Autodesk Fusion 360 part; units mm, degrees
(part 4 of 6)
sketch "USB clamp fixed housing post sketch" plane through (0, 0, 37.2) normal (0, 0, 1) x (1, 0, 0) in component "01 Tapered printed housing"
  circle A0 centre (70, 16) radius 4.3
  dimension "d1306" = 70
  dimension "d1307" = 16
  dimension "d1308" = 4.3
  measures "d1306" horizontal distance of origin A0.centre
  measures "d1307" vertical distance of origin A0.centre
  measures "d1308" radius of A0
extrude "USB clamp fixed housing post" add sketch "USB clamp fixed housing post sketch" along normal blind 6 bodies 1 in component "01 Tapered printed housing"
ref_plane "WorkPlane33" through (0, 0, 39.2) normal (0, 0, 1) x (1, 0, 0) in component "01 Tapered printed housing"
sketch "USB clamp insert pilot reference sketch" plane through (0, 0, 39.2) normal (0, 0, 1) x (1, 0, 0) in component "01 Tapered printed housing"
  circle A0 centre (69.3, 16) radius 1.6
  dimension "d1313" = 69.3
  dimension "d1314" = 16
  dimension "d1315" = 1.6
  measures "d1313" horizontal distance of origin A0.centre
  measures "d1314" vertical distance of origin A0.centre
  measures "d1315" radius of A0
extrude "USB clamp insert pilot reference" cut sketch "USB clamp insert pilot reference sketch" along normal blind 4.1 bodies 1 in component "01 Tapered printed housing"
ref_plane "WorkPlane1" through (0, 0, 43.2) normal (0, 0, 1) x (1, 0, 0) in component "USB — removable rear housing clamp"
sketch "USB rear clamp strap sketch" plane through (0, 0, 43.2) normal (0, 0, 1) x (1, 0, 0) in component "USB — removable rear housing clamp"
  line L0 (65.7, 8.5) -> (72.4, 8.5)
  line L1 (72.4, 8.5) -> (72.4, 20.3)
  line L2 (72.4, 20.3) -> (65.7, 20.3)
  line L3 (65.7, 20.3) -> (65.7, 8.5)
  dimension "d1320" = 65.7
  dimension "d1321" = 8.5
  dimension "d1322" = 6.7
  dimension "d1323" = 11.8
  constraint horizontal L0
  constraint vertical L1
  constraint horizontal L2
  constraint vertical L3
  measures "d1320" horizontal distance of origin L0.start
  measures "d1321" vertical distance of origin L0.start
  measures "d1322" horizontal distance of L0.start L0.end
  measures "d1323" vertical distance of L0.end L1.end
extrude "USB rear clamp strap" add sketch "USB rear clamp strap sketch" along normal blind 2 separate body makes body 61 in component "USB — removable rear housing clamp"
ref_plane "WorkPlane2" through (0, 0, 35) normal (0, 0, 1) x (1, 0, 0) in component "USB — removable rear housing clamp"
sketch "USB inward stop and offset stalk sketch" plane through (0, 0, 35) normal (0, 0, 1) x (1, 0, 0) in component "USB — removable rear housing clamp"
  line L0 (68.4, 8.5) -> (70.4, 8.5)
  line L1 (70.4, 8.5) -> (70.4, 10.5)
  line L2 (70.4, 10.5) -> (68.4, 10.5)
  line L3 (68.4, 10.5) -> (68.4, 8.5)
  dimension "d1328" = 68.4
  dimension "d1329" = 8.5
  dimension "d1330" = 2
  dimension "d1331" = 2
  constraint horizontal L0
  constraint vertical L1
  constraint horizontal L2
  constraint vertical L3
  measures "d1328" horizontal distance of origin L0.start
  measures "d1329" vertical distance of origin L0.start
  measures "d1330" horizontal distance of L0.start L0.end
  measures "d1331" vertical distance of L0.end L1.end
extrude "USB inward stop and offset stalk" add sketch "USB inward stop and offset stalk sketch" along normal blind 8.3 bodies 61 in component "USB — removable rear housing clamp"
ref_plane "WorkPlane3" through (0, 0, 43.1) normal (0, 0, 1) x (1, 0, 0) in component "USB — removable rear housing clamp"
sketch "USB clamp M2 clearance sketch" plane through (0, 0, 43.1) normal (0, 0, 1) x (1, 0, 0) in component "USB — removable rear housing clamp"
  circle A0 centre (69.3, 16) radius 1.1
  dimension "d1336" = 69.3
  dimension "d1337" = 16
  dimension "d1338" = 1.1
  measures "d1336" horizontal distance of origin A0.centre
  measures "d1337" vertical distance of origin A0.centre
  measures "d1338" radius of A0
extrude "USB clamp M2 clearance" cut sketch "USB clamp M2 clearance sketch" along normal blind 2.2 bodies 61 in component "USB — removable rear housing clamp"
ref_plane "WorkPlane1" through (0, 0, 48.8) normal (0, 0, 1) x (1, 0, 0) in component "Chamber / removable internal lid"
sketch "Internal L lid sketch" plane through (0, 0, 48.8) normal (0, 0, 1) x (1, 0, 0) in component "Chamber / removable internal lid"
  line L0 (2.9, 87) -> (72.1, 87)
  line L1 (72.1, 87) -> (72.1, 122.1)
  line L2 (72.1, 122.1) -> (2.9, 122.1)
  line L3 (2.9, 122.1) -> (2.9, 87)
  dimension "d1609" = 2.9
  dimension "d1610" = 87
  constraint horizontal L0
  constraint vertical L1
  constraint horizontal L2
  constraint vertical L3
  measures "d1609" horizontal distance of origin L0.start
  measures "d1610" vertical distance of origin L0.start
extrude "Internal L lid" add sketch "Internal L lid sketch" along normal blind 2 separate body makes body 62 in component "Chamber / removable internal lid"
ref_plane "WorkPlane2" through (0, 0, 48.8) normal (0, 0, 1) x (1, 0, 0) in component "Chamber / removable internal lid"
sketch "Internal L lid side column sketch" plane through (0, 0, 48.8) normal (0, 0, 1) x (1, 0, 0) in component "Chamber / removable internal lid"
  line L0 (45.6, 30) -> (72.1, 30)
  line L1 (72.1, 30) -> (72.1, 122.1)
  line L2 (72.1, 122.1) -> (45.6, 122.1)
  line L3 (45.6, 122.1) -> (45.6, 30)
  dimension "d1617" = 45.6
  dimension "d1618" = 30
  constraint horizontal L0
  constraint vertical L1
  constraint horizontal L2
  constraint vertical L3
  measures "d1617" horizontal distance of origin L0.start
  measures "d1618" vertical distance of origin L0.start
extrude "Internal L lid side column" add sketch "Internal L lid side column sketch" along normal blind 2 bodies 62 in component "Chamber / removable internal lid"
fillet "Lid housing-clearance top rounds" radius 3.1 2 edges at (2.9, 122.1, 49.8) (72.1, 122.1, 49.8) on bodies 62 in component "Chamber / removable internal lid"
ref_plane "WorkPlane3" through (0, 0, 15.5) normal (0, 0, 1) x (1, 0, 0) in component "Chamber / removable internal lid"
sketch "Lid upper M3 post clearance sketch" plane through (0, 0, 15.5) normal (0, 0, 1) x (1, 0, 0) in component "Chamber / removable internal lid"
  circle A0 centre (6, 119) radius 4.5
  dimension "d1627" = 6
  dimension "d1628" = 119
  dimension "d1629" = 4.5
  measures "d1627" horizontal distance of origin A0.centre
  measures "d1628" vertical distance of origin A0.centre
  measures "d1629" radius of A0
extrude "Lid upper M3 post clearance" cut sketch "Lid upper M3 post clearance sketch" along normal blind 112 bodies 62 in component "Chamber / removable internal lid"
ref_plane "WorkPlane4" through (0, 0, 15.5) normal (0, 0, 1) x (1, 0, 0) in component "Chamber / removable internal lid"
sketch "Lid upper M3 post clearance sketch (1)" plane through (0, 0, 15.5) normal (0, 0, 1) x (1, 0, 0) in component "Chamber / removable internal lid"
  circle A0 centre (69, 119) radius 4.5
  dimension "d1634" = 69
  dimension "d1635" = 119
  dimension "d1636" = 4.5
  measures "d1634" horizontal distance of origin A0.centre
  measures "d1635" vertical distance of origin A0.centre
  measures "d1636" radius of A0
extrude "Lid upper M3 post clearance (1)" cut sketch "Lid upper M3 post clearance sketch (1)" along normal blind 112 bodies 62 in component "Chamber / removable internal lid"
ref_plane "WorkPlane5" through (0, 0, 15.5) normal (0, 0, 1) x (1, 0, 0) in component "Chamber / removable internal lid"
sketch "Lid upper display retainer service notch sketch" plane through (0, 0, 15.5) normal (0, 0, 1) x (1, 0, 0) in component "Chamber / removable internal lid"
  line L0 (1.9, 114.8) -> (18.1, 114.8)
  line L1 (18.1, 114.8) -> (18.1, 125)
  line L2 (18.1, 125) -> (1.9, 125)
  line L3 (1.9, 125) -> (1.9, 114.8)
  dimension "d1641" = 1.9
  dimension "d1642" = 114.8
  dimension "d1643" = 16.2
  dimension "d1644" = 10.2
  constraint horizontal L0
  constraint vertical L1
  constraint horizontal L2
  constraint vertical L3
  measures "d1641" horizontal distance of origin L0.start
  measures "d1642" vertical distance of origin L0.start
  measures "d1643" horizontal distance of L0.start L0.end
  measures "d1644" vertical distance of L0.end L1.end
extrude "Lid upper display retainer service notch" cut sketch "Lid upper display retainer service notch sketch" along normal blind 112 bodies 62 in component "Chamber / removable internal lid"
ref_plane "WorkPlane6" through (0, 0, 48.7) normal (0, 0, 1) x (1, 0, 0) in component "Chamber / removable internal lid"
sketch "Internal lid M2 clearance sketch" plane through (0, 0, 48.7) normal (0, 0, 1) x (1, 0, 0) in component "Chamber / removable internal lid"
  circle A0 centre (17.4, 92.6) radius 1.2
  dimension "d1649" = 17.4
  dimension "d1650" = 92.6
  dimension "d1651" = 1.2
  measures "d1649" horizontal distance of origin A0.centre
  measures "d1650" vertical distance of origin A0.centre
  measures "d1651" radius of A0
extrude "Internal lid M2 clearance" cut sketch "Internal lid M2 clearance sketch" along normal blind 2.2 bodies 62 in component "Chamber / removable internal lid"
ref_plane "WorkPlane7" through (0, 0, 48.7) normal (0, 0, 1) x (1, 0, 0) in component "Chamber / removable internal lid"
sketch "Internal lid M2 clearance sketch (1)" plane through (0, 0, 48.7) normal (0, 0, 1) x (1, 0, 0) in component "Chamber / removable internal lid"
  circle A0 centre (12.9, 110.6) radius 1.2
  dimension "d1656" = 12.9
  dimension "d1657" = 110.6
  dimension "d1658" = 1.2
  measures "d1656" horizontal distance of origin A0.centre
  measures "d1657" vertical distance of origin A0.centre
  measures "d1658" radius of A0
extrude "Internal lid M2 clearance (1)" cut sketch "Internal lid M2 clearance sketch (1)" along normal blind 2.2 bodies 62 in component "Chamber / removable internal lid"
ref_plane "WorkPlane8" through (0, 0, 48.7) normal (0, 0, 1) x (1, 0, 0) in component "Chamber / removable internal lid"
sketch "Internal lid M2 clearance sketch (2)" plane through (0, 0, 48.7) normal (0, 0, 1) x (1, 0, 0) in component "Chamber / removable internal lid"
  circle A0 centre (66.5, 83.5) radius 1.2
  dimension "d1663" = 66.5
  dimension "d1664" = 83.5
  dimension "d1665" = 1.2
  measures "d1663" horizontal distance of origin A0.centre
  measures "d1664" vertical distance of origin A0.centre
  measures "d1665" radius of A0
extrude "Internal lid M2 clearance (2)" cut sketch "Internal lid M2 clearance sketch (2)" along normal blind 2.2 bodies 62 in component "Chamber / removable internal lid"
ref_plane "WorkPlane9" through (0, 0, 48.7) normal (0, 0, 1) x (1, 0, 0) in component "Chamber / removable internal lid"
sketch "Internal lid M2 clearance sketch (3)" plane through (0, 0, 48.7) normal (0, 0, 1) x (1, 0, 0) in component "Chamber / removable internal lid"
  circle A0 centre (66.5, 110.5) radius 1.2
  dimension "d1670" = 66.5
  dimension "d1671" = 110.5
  dimension "d1672" = 1.2
  measures "d1670" horizontal distance of origin A0.centre
  measures "d1671" vertical distance of origin A0.centre
  measures "d1672" radius of A0
extrude "Internal lid M2 clearance (3)" cut sketch "Internal lid M2 clearance sketch (3)" along normal blind 2.2 bodies 62 in component "Chamber / removable internal lid"
ref_plane "WorkPlane10" through (0, 0, 48.7) normal (0, 0, 1) x (1, 0, 0) in component "Chamber / removable internal lid"
sketch "Internal lid M2 clearance sketch (4)" plane through (0, 0, 48.7) normal (0, 0, 1) x (1, 0, 0) in component "Chamber / removable internal lid"
  circle A0 centre (51.2, 34) radius 1.2
  dimension "d1677" = 51.2
  dimension "d1678" = 34
  dimension "d1679" = 1.2
  measures "d1677" horizontal distance of origin A0.centre
  measures "d1678" vertical distance of origin A0.centre
  measures "d1679" radius of A0
extrude "Internal lid M2 clearance (4)" cut sketch "Internal lid M2 clearance sketch (4)" along normal blind 2.2 bodies 62 in component "Chamber / removable internal lid"
ref_plane "WorkPlane11" through (0, 0, 48.7) normal (0, 0, 1) x (1, 0, 0) in component "Chamber / removable internal lid"
sketch "Internal lid M2 clearance sketch (5)" plane through (0, 0, 48.7) normal (0, 0, 1) x (1, 0, 0) in component "Chamber / removable internal lid"
  circle A0 centre (66.5, 34) radius 1.2
  dimension "d1684" = 66.5
  dimension "d1685" = 34
  dimension "d1686" = 1.2
  measures "d1684" horizontal distance of origin A0.centre
  measures "d1685" vertical distance of origin A0.centre
  measures "d1686" radius of A0
extrude "Internal lid M2 clearance (5)" cut sketch "Internal lid M2 clearance sketch (5)" along normal blind 2.2 bodies 62 in component "Chamber / removable internal lid"
ref_plane "WorkPlane12" through (0, 0, 48.7) normal (0, 0, 1) x (1, 0, 0) in component "Chamber / removable internal lid"
sketch "Mounting screw driver access inside isolated tunnel sketch" plane through (0, 0, 48.7) normal (0, 0, 1) x (1, 0, 0) in component "Chamber / removable internal lid"
  circle A0 centre (8.8, 94.7) radius 2.7
  dimension "d1691" = 8.8
  dimension "d1692" = 94.7
  dimension "d1693" = 2.7
  measures "d1691" horizontal distance of origin A0.centre
  measures "d1692" vertical distance of origin A0.centre
  measures "d1693" radius of A0
extrude "Mounting screw driver access inside isolated tunnel" cut sketch "Mounting screw driver access inside isolated tunnel sketch" along normal blind 2.2 bodies 62 in component "Chamber / removable internal lid"
ref_plane "WorkPlane13" through (0, 0, 48.7) normal (0, 0, 1) x (1, 0, 0) in component "Chamber / removable internal lid"
sketch "Mounting screw driver access inside isolated tunnel sketch (1)" plane through (0, 0, 48.7) normal (0, 0, 1) x (1, 0, 0) in component "Chamber / removable internal lid"
  circle A0 centre (59.2, 115.4) radius 2.7
  dimension "d1698" = 59.2
  dimension "d1699" = 115.4
  dimension "d1700" = 2.7
  measures "d1698" horizontal distance of origin A0.centre
  measures "d1699" vertical distance of origin A0.centre
  measures "d1700" radius of A0
extrude "Mounting screw driver access inside isolated tunnel (1)" cut sketch "Mounting screw driver access inside isolated tunnel sketch (1)" along normal blind 2.2 bodies 62 in component "Chamber / removable internal lid"
ref_plane "WorkPlane34" through (0, 0, 14.3) normal (0, 0, 1) x (1, 0, 0) in component "01 Tapered printed housing"
sketch "Left cartridge post front support bridge sketch" plane through (0, 0, 14.3) normal (0, 0, 1) x (1, 0, 0) in component "01 Tapered printed housing"
  line L0 (2.1, 91.05) -> (8.8, 91.05)
  line L1 (8.8, 91.05) -> (8.8, 98.35)
  line L2 (8.8, 98.35) -> (2.1, 98.35)
  line L3 (2.1, 98.35) -> (2.1, 91.05)
  dimension "d1705" = 2.1
  dimension "d1706" = 91.05
  dimension "d1707" = 6.7
  dimension "d1708" = 7.3
  constraint horizontal L0
  constraint vertical L1
  constraint horizontal L2
  constraint vertical L3
  measures "d1705" horizontal distance of origin L0.start
  measures "d1706" vertical distance of origin L0.start
  measures "d1707" horizontal distance of L0.start L0.end
  measures "d1708" vertical distance of L0.end L1.end
extrude "Left cartridge post front support bridge" add sketch "Left cartridge post front support bridge sketch" along normal blind 2 bodies 1 in component "01 Tapered printed housing"
ref_plane "WorkPlane35" through (0, 0, 14.3) normal (0, 0, 1) x (1, 0, 0) in component "01 Tapered printed housing"
sketch "Top cartridge post front support bridge sketch" plane through (0, 0, 14.3) normal (0, 0, 1) x (1, 0, 0) in component "01 Tapered printed housing"
  line L0 (55.55, 115.4) -> (62.85, 115.4)
  line L1 (62.85, 115.4) -> (62.85, 122.9)
  line L2 (62.85, 122.9) -> (55.55, 122.9)
  line L3 (55.55, 122.9) -> (55.55, 115.4)
  dimension "d1713" = 55.55
  dimension "d1714" = 115.4
  dimension "d1715" = 7.3
  dimension "d1716" = 7.5
  constraint horizontal L0
  constraint vertical L1
  constraint horizontal L2
  constraint vertical L3
  measures "d1713" horizontal distance of origin L0.start
  measures "d1714" vertical distance of origin L0.start
  measures "d1715" horizontal distance of L0.start L0.end
  measures "d1716" vertical distance of L0.end L1.end
extrude "Top cartridge post front support bridge" add sketch "Top cartridge post front support bridge sketch" along normal blind 2 bodies 1 in component "01 Tapered printed housing"
ref_plane "WorkPlane36" through (0, 0, 14.3) normal (0, 0, 1) x (1, 0, 0) in component "01 Tapered printed housing"
sketch "Stationary isolated cartridge M2 post sketch" plane through (0, 0, 14.3) normal (0, 0, 1) x (1, 0, 0) in component "01 Tapered printed housing"
  circle A0 centre (8.8, 94.7) radius 3.65
  dimension "d1721" = 8.8
  dimension "d1722" = 94.7
  dimension "d1723" = 3.65
  measures "d1721" horizontal distance of origin A0.centre
  measures "d1722" vertical distance of origin A0.centre
  measures "d1723" radius of A0
extrude "Stationary isolated cartridge M2 post" add sketch "Stationary isolated cartridge M2 post sketch" along normal blind 32.5 bodies 1 in component "01 Tapered printed housing"
ref_plane "WorkPlane37" through (0, 0, 42.8) normal (0, 0, 1) x (1, 0, 0) in component "01 Tapered printed housing"
sketch "Cartridge mount insert pocket sketch" plane through (0, 0, 42.8) normal (0, 0, 1) x (1, 0, 0) in component "01 Tapered printed housing"
  circle A0 centre (8.8, 94.7) radius 1.65
  dimension "d1728" = 8.8
  dimension "d1729" = 94.7
  dimension "d1730" = 1.65
  measures "d1728" horizontal distance of origin A0.centre
  measures "d1729" vertical distance of origin A0.centre
  measures "d1730" radius of A0
extrude "Cartridge mount insert pocket" cut sketch "Cartridge mount insert pocket sketch" along normal blind 4.1 bodies 1 in component "01 Tapered printed housing"
ref_plane "WorkPlane38" through (0, 0, 14.3) normal (0, 0, 1) x (1, 0, 0) in component "01 Tapered printed housing"
sketch "Stationary isolated cartridge M2 post sketch (1)" plane through (0, 0, 14.3) normal (0, 0, 1) x (1, 0, 0) in component "01 Tapered printed housing"
  circle A0 centre (59.2, 115.4) radius 3.65
  dimension "d1735" = 59.2
  dimension "d1736" = 115.4
  dimension "d1737" = 3.65
  measures "d1735" horizontal distance of origin A0.centre
  measures "d1736" vertical distance of origin A0.centre
  measures "d1737" radius of A0
extrude "Stationary isolated cartridge M2 post (1)" add sketch "Stationary isolated cartridge M2 post sketch (1)" along normal blind 32.5 bodies 1 in component "01 Tapered printed housing"
ref_plane "WorkPlane39" through (0, 0, 42.8) normal (0, 0, 1) x (1, 0, 0) in component "01 Tapered printed housing"
sketch "Cartridge mount insert pocket sketch (1)" plane through (0, 0, 42.8) normal (0, 0, 1) x (1, 0, 0) in component "01 Tapered printed housing"
  circle A0 centre (59.2, 115.4) radius 1.65
  dimension "d1742" = 59.2
  dimension "d1743" = 115.4
  dimension "d1744" = 1.65
  measures "d1742" horizontal distance of origin A0.centre
  measures "d1743" vertical distance of origin A0.centre
  measures "d1744" radius of A0
extrude "Cartridge mount insert pocket (1)" cut sketch "Cartridge mount insert pocket sketch (1)" along normal blind 4.1 bodies 1 in component "01 Tapered printed housing"
ref_plane "WorkPlane1" through (21.4, 0, 0) normal (1, 0, 0) x (0, 1, 0) in component "Sensor / AO2 sideways body and neck"
sketch "AO2 full-size body sketch" plane through (21.4, 0, 0) normal (1, 0, 0) x (0, 0, -1) in component "Sensor / AO2 sideways body and neck"
  circle A0 centre (-33.65, 104.3) radius 14.65
  dimension "d1749" = 33.65
  dimension "d1750" = 104.3
  dimension "d1751" = 14.65
  measures "d1749" horizontal distance of origin A0.centre
  measures "d1750" vertical distance of origin A0.centre
  measures "d1751" radius of A0
extrude "AO2 full-size body" add sketch "AO2 full-size body sketch" along normal blind 31.75 separate body makes body 63 in component "Sensor / AO2 sideways body and neck"
ref_plane "WorkPlane2" through (14.9, 0, 0) normal (1, 0, 0) x (0, 1, 0) in component "Sensor / AO2 sideways body and neck"
sketch "AO2 M16 nose reference sketch" plane through (14.9, 0, 0) normal (1, 0, 0) x (0, 0, -1) in component "Sensor / AO2 sideways body and neck"
  circle A0 centre (-33.65, 104.3) radius 8
  dimension "d1756" = 33.65
  dimension "d1757" = 104.3
  dimension "d1758" = 8
  measures "d1756" horizontal distance of origin A0.centre
  measures "d1757" vertical distance of origin A0.centre
  measures "d1758" radius of A0
extrude "AO2 M16 nose reference" add sketch "AO2 M16 nose reference sketch" along normal blind 6.5 bodies 63 in component "Sensor / AO2 sideways body and neck"
ref_plane "WorkPlane1" through (0, 0, 28.65) normal (0, 0, 1) x (1, 0, 0) in component "Sensor / AO2 connector allowance"
sketch "AO2 connector allowance sketch" plane through (0, 0, 28.65) normal (0, 0, 1) x (1, 0, 0) in component "Sensor / AO2 connector allowance"
  line L0 (53.15, 99.3) -> (59.65, 99.3)
  line L1 (59.65, 99.3) -> (59.65, 109.3)
  line L2 (59.65, 109.3) -> (53.15, 109.3)
  line L3 (53.15, 109.3) -> (53.15, 99.3)
  dimension "d1763" = 53.15
  dimension "d1764" = 99.3
  dimension "d1765" = 6.5
  dimension "d1766" = 10
  constraint horizontal L0
  constraint vertical L1
  constraint horizontal L2
  constraint vertical L3
  measures "d1763" horizontal distance of origin L0.start
  measures "d1764" vertical distance of origin L0.start
  measures "d1765" horizontal distance of L0.start L0.end
  measures "d1766" vertical distance of L0.end L1.end
extrude "AO2 connector allowance" add sketch "AO2 connector allowance sketch" along normal blind 10 separate body makes body 64 in component "Sensor / AO2 connector allowance"
ref_plane "WorkPlane1" through (0, 0, 19) normal (0, 0, 1) x (1, 0, 0) in component "Sensor / ZE07-CO rotated total envelope"
sketch "ZE07-CO rotated total envelope sketch" plane through (0, 0, 19) normal (0, 0, 1) x (1, 0, 0) in component "Sensor / ZE07-CO rotated total envelope"
  line L0 (47.975, 38) -> (69.725, 38)
  line L1 (69.725, 38) -> (69.725, 60.4)
  line L2 (69.725, 60.4) -> (47.975, 60.4)
  line L3 (47.975, 60.4) -> (47.975, 38)
  dimension "d1771" = 47.975
  dimension "d1772" = 38
  dimension "d1773" = 21.75
  dimension "d1774" = 22.4
  constraint horizontal L0
  constraint vertical L1
  constraint horizontal L2
  constraint vertical L3
  measures "d1771" horizontal distance of origin L0.start
  measures "d1772" vertical distance of origin L0.start
  measures "d1773" horizontal distance of L0.start L0.end
  measures "d1774" vertical distance of L0.end L1.end
extrude "ZE07-CO rotated total envelope" add sketch "ZE07-CO rotated total envelope sketch" along normal blind 25.4 separate body makes body 65 in component "Sensor / ZE07-CO rotated total envelope"
ref_plane "WorkPlane1" through (0, 0, 19) normal (0, 0, 1) x (1, 0, 0) in component "Sensor / MD62 rotated body envelope"
sketch "MD62 rotated body envelope sketch" plane through (0, 0, 19) normal (0, 0, 1) x (1, 0, 0) in component "Sensor / MD62 rotated body envelope"
  line L0 (60.1, 61) -> (69.6, 61)
  line L1 (69.6, 61) -> (69.6, 75)
  line L2 (69.6, 75) -> (60.1, 75)
  line L3 (60.1, 75) -> (60.1, 61)
  dimension "d1779" = 60.1
  dimension "d1780" = 61
  dimension "d1781" = 9.5
  dimension "d1782" = 14
  constraint horizontal L0
  constraint vertical L1
  constraint horizontal L2
  constraint vertical L3
  measures "d1779" horizontal distance of origin L0.start
  measures "d1780" vertical distance of origin L0.start
  measures "d1781" horizontal distance of L0.start L0.end
  measures "d1782" vertical distance of L0.end L1.end
extrude "MD62 rotated body envelope" add sketch "MD62 rotated body envelope sketch" along normal blind 19 separate body makes body 66 in component "Sensor / MD62 rotated body envelope"
ref_plane "WorkPlane1" through (0, 0, 19) normal (0, 0, 1) x (1, 0, 0) in component "Sensor / MD62 27 mm lead allowance"
sketch "MD62 27 mm lead allowance sketch" plane through (0, 0, 19) normal (0, 0, 1) x (1, 0, 0) in component "Sensor / MD62 27 mm lead allowance"
  line L0 (60.1, 75) -> (69.6, 75)
  line L1 (69.6, 75) -> (69.6, 102)
  line L2 (69.6, 102) -> (60.1, 102)
  line L3 (60.1, 102) -> (60.1, 75)
  dimension "d1787" = 60.1
  dimension "d1788" = 75
  dimension "d1789" = 9.5
  dimension "d1790" = 27
  constraint horizontal L0
  constraint vertical L1
  constraint horizontal L2
  constraint vertical L3
  measures "d1787" horizontal distance of origin L0.start
  measures "d1788" vertical distance of origin L0.start
  measures "d1789" horizontal distance of L0.start L0.end
  measures "d1790" vertical distance of L0.end L1.end
extrude "MD62 27 mm lead allowance" add sketch "MD62 27 mm lead allowance sketch" along normal blind 19 separate body makes body 67 in component "Sensor / MD62 27 mm lead allowance"
ref_plane "WorkPlane1" through (0, 0, 42) normal (0, 0, 1) x (1, 0, 0) in component "Sensor / GYBMEP wired module envelope"
sketch "GYBMEP wired module envelope sketch" plane through (0, 0, 42) normal (0, 0, 1) x (1, 0, 0) in component "Sensor / GYBMEP wired module envelope"
  line L0 (55.5, 88.8) -> (67.5, 88.8)
  line L1 (67.5, 88.8) -> (67.5, 105.8)
  line L2 (67.5, 105.8) -> (55.5, 105.8)
  line L3 (55.5, 105.8) -> (55.5, 88.8)
  dimension "d1795" = 55.5
  dimension "d1796" = 88.8
  dimension "d1797" = 12
  dimension "d1798" = 17
  constraint horizontal L0
  constraint vertical L1
  constraint horizontal L2
  constraint vertical L3
  measures "d1795" horizontal distance of origin L0.start
  measures "d1796" vertical distance of origin L0.start
  measures "d1797" horizontal distance of L0.start L0.end
  measures "d1798" vertical distance of L0.end L1.end
extrude "GYBMEP wired module envelope" add sketch "GYBMEP wired module envelope sketch" along normal blind 5 separate body makes body 68 in component "Sensor / GYBMEP wired module envelope"
ref_plane "WorkPlane1" through (70.1, 0, 0) normal (1, 0, 0) x (0, 1, 0) in component "Gas / left inlet fitting reference"
sketch "left inlet hollow fitting sketch" plane through (70.1, 0, 0) normal (1, 0, 0) x (0, 0, -1) in component "Gas / left inlet fitting reference"
  circle A0 centre (-23, 105) radius 4
  dimension "d1804" = 105
  dimension "d1805" = 4
  measures "d1804" vertical distance of origin A0.centre
  measures "d1805" radius of A0
extrude "left inlet hollow fitting" add sketch "left inlet hollow fitting sketch" along normal blind 10.9 separate body makes body 69 in component "Gas / left inlet fitting reference"
ref_plane "WorkPlane2" through (70, 0, 0) normal (1, 0, 0) x (0, 1, 0) in component "Gas / left inlet fitting reference"
sketch "left inlet 5 mm through bore sketch" plane through (70, 0, 0) normal (1, 0, 0) x (0, 0, -1) in component "Gas / left inlet fitting reference"
  circle A0 centre (-23, 105) radius 2.5
  dimension "d1811" = 105
  dimension "d1812" = 2.5
  measures "d1811" vertical distance of origin A0.centre
  measures "d1812" radius of A0
extrude "left inlet 5 mm through bore" cut sketch "left inlet 5 mm through bore sketch" along normal blind 11.1 bodies 69 in component "Gas / left inlet fitting reference"
ref_plane "WorkPlane1" through (-6, 0, 0) normal (1, 0, 0) x (0, 1, 0) in component "Gas / right exhaust fitting reference"
sketch "right exhaust hollow fitting sketch" plane through (-6, 0, 0) normal (1, 0, 0) x (0, 0, -1) in component "Gas / right exhaust fitting reference"
  circle A0 centre (-23, 105) radius 4
  dimension "d1818" = 105
  dimension "d1819" = 4
  measures "d1818" vertical distance of origin A0.centre
  measures "d1819" radius of A0
extrude "right exhaust hollow fitting" add sketch "right exhaust hollow fitting sketch" along normal blind 10.9 separate body makes body 70 in component "Gas / right exhaust fitting reference"
ref_plane "WorkPlane2" through (-6.1, 0, 0) normal (1, 0, 0) x (0, 1, 0) in component "Gas / right exhaust fitting reference"
sketch "right exhaust 5 mm through bore sketch" plane through (-6.1, 0, 0) normal (1, 0, 0) x (0, 0, -1) in component "Gas / right exhaust fitting reference"
  circle A0 centre (-23, 105) radius 2.5
  dimension "d1825" = 105
  dimension "d1826" = 2.5
  measures "d1825" vertical distance of origin A0.centre
  measures "d1826" radius of A0
extrude "right exhaust 5 mm through bore" cut sketch "right exhaust 5 mm through bore sketch" along normal blind 11.1 bodies 70 in component "Gas / right exhaust fitting reference"
ref_plane "WorkPlane1" through (42, 0, 0) normal (1, 0, 0) x (0, 1, 0) in component "Chamber / sealed wire feedthrough concept"
sketch "Harness feedthrough envelope sketch" plane through (42, 0, 0) normal (1, 0, 0) x (0, 0, -1) in component "Chamber / sealed wire feedthrough concept"
  circle A0 centre (-44.5, 73) radius 2.2
  dimension "d1831" = 44.5
  dimension "d1832" = 73
  dimension "d1833" = 2.2
  measures "d1831" horizontal distance of origin A0.centre
  measures "d1832" vertical distance of origin A0.centre
  measures "d1833" radius of A0
extrude "Harness feedthrough envelope" add sketch "Harness feedthrough envelope sketch" along normal blind 5.6 separate body makes body 71 in component "Chamber / sealed wire feedthrough concept"
ref_plane "WorkPlane2" through (41.9, 0, 0) normal (1, 0, 0) x (0, 1, 0) in component "Chamber / sealed wire feedthrough concept"
sketch "Sketch2 (3)" plane through (41.9, 0, 0) normal (1, 0, 0) x (0, 0, -1) in component "Chamber / sealed wire feedthrough concept"
  circle A0 centre (-44.5, 73) radius 1.3
  dimension "d1838" = 44.5
  dimension "d1839" = 73
  dimension "d1840" = 1.3
  measures "d1838" horizontal distance of origin A0.centre
  measures "d1839" vertical distance of origin A0.centre
  measures "d1840" radius of A0
extrude "Provisional wire bore — sealing pending" cut sketch "Sketch2 (3)" along normal blind 5.8 bodies 71 in component "Chamber / sealed wire feedthrough concept"
delete_body "RemoveBody1" bodies 65 in component "Sensor / ZE07-CO rotated total envelope"
ref_plane "WorkPlane2" through (0, 0, 19) normal (0, 0, 1) x (1, 0, 0) in component "Sensor / ZE07-CO rotated total envelope"
sketch "Sketch2 (4)" plane through (0, 0, 19) normal (0, 0, 1) x (1, 0, 0) in component "Sensor / ZE07-CO rotated total envelope"
  line L0 (51.425, 38) -> (53.025, 38)
  line L1 (53.025, 38) -> (53.025, 60.4)
  line L2 (53.025, 60.4) -> (51.425, 60.4)
  line L3 (51.425, 60.4) -> (51.425, 38)
  dimension "d1845" = 51.425
  dimension "d1846" = 38
  dimension "d1847" = 1.6
  dimension "d1848" = 22.4
  constraint horizontal L0
  constraint vertical L1
  constraint horizontal L2
  constraint vertical L3
  measures "d1845" horizontal distance of origin L0.start
  measures "d1846" vertical distance of origin L0.start
  measures "d1847" horizontal distance of L0.start L0.end
  measures "d1848" vertical distance of L0.end L1.end
extrude "ZE07-CO PCB — drawing-derived stack" add sketch "Sketch2 (4)" along normal blind 25.4 separate body makes body 72 in component "Sensor / ZE07-CO rotated total envelope"
ref_plane "WorkPlane3" through (53.025, 0, 0) normal (1, 0, 0) x (0, 1, 0) in component "Sensor / ZE07-CO rotated total envelope"
sketch "Sketch3 (2)" plane through (53.025, 0, 0) normal (1, 0, 0) x (0, 0, -1) in component "Sensor / ZE07-CO rotated total envelope"
  circle A0 centre (-31.7, 49.2) radius 10
  dimension "d1853" = 31.7
  dimension "d1854" = 49.2
  dimension "d1855" = 10
  measures "d1853" horizontal distance of origin A0.centre
  measures "d1854" vertical distance of origin A0.centre
  measures "d1855" radius of A0
extrude "ZE07-CO sensor can — Ø20 x 16.7 reference" add sketch "Sketch3 (2)" along normal blind 16.7 separate body makes body 73 in component "Sensor / ZE07-CO rotated total envelope"
ref_plane "WorkPlane4" through (0, 0, 27.5) normal (0, 0, 1) x (1, 0, 0) in component "Sensor / ZE07-CO rotated total envelope"
sketch "Sketch4 (2)" plane through (0, 0, 27.5) normal (0, 0, 1) x (1, 0, 0) in component "Sensor / ZE07-CO rotated total envelope"
  line L0 (47.975, 40) -> (51.425, 40)
  line L1 (51.425, 40) -> (51.425, 46)
  line L2 (51.425, 46) -> (47.975, 46)
  line L3 (47.975, 46) -> (47.975, 40)
  dimension "d1860" = 47.975
  dimension "d1861" = 40
  dimension "d1862" = 3.45
  dimension "d1863" = 6
  constraint horizontal L0
  constraint vertical L1
  constraint horizontal L2
  constraint vertical L3
  measures "d1860" horizontal distance of origin L0.start
  measures "d1861" vertical distance of origin L0.start
  measures "d1862" horizontal distance of L0.start L0.end
  measures "d1863" vertical distance of L0.end L1.end
extrude "ZE07 opposite-side pin header allowance — profile unmeasured" add sketch "Sketch4 (2)" along normal blind 8 separate body makes body 74 in component "Sensor / ZE07-CO rotated total envelope"
delete_body "RemoveBody1'" bodies 68 in component "Sensor / GYBMEP wired module envelope"
ref_plane "WorkPlane2" through (0, 0, 42) normal (0, 0, 1) x (1, 0, 0) in component "Sensor / GYBMEP wired module envelope"
sketch "Sketch2 (5)" plane through (0, 0, 42) normal (0, 0, 1) x (1, 0, 0) in component "Sensor / GYBMEP wired module envelope"
  line L0 (55.5, 88.8) -> (67.5, 88.8)
  line L1 (67.5, 88.8) -> (67.5, 105.8)
  line L2 (67.5, 105.8) -> (55.5, 105.8)
  line L3 (55.5, 105.8) -> (55.5, 88.8)
  dimension "d1868" = 55.5
  dimension "d1869" = 88.8
  dimension "d1870" = 12
  dimension "d1871" = 17
  constraint horizontal L0
  constraint vertical L1
  constraint horizontal L2
  constraint vertical L3
  measures "d1868" horizontal distance of origin L0.start
  measures "d1869" vertical distance of origin L0.start
  measures "d1870" horizontal distance of L0.start L0.end
  measures "d1871" vertical distance of L0.end L1.end
extrude "GYBMEP board — provisional visual reference" add sketch "Sketch2 (5)" along normal blind 1.6 separate body makes body 75 in component "Sensor / GYBMEP wired module envelope"
ref_plane "WorkPlane3" through (0, 0, 41.9) normal (0, 0, 1) x (1, 0, 0) in component "Sensor / GYBMEP wired module envelope"
sketch "Sketch3 (3)" plane through (0, 0, 41.9) normal (0, 0, 1) x (1, 0, 0) in component "Sensor / GYBMEP wired module envelope"
  circle A0 centre (57.2, 90.3) radius 0.5
  dimension "d1876" = 57.2
  dimension "d1877" = 90.3
  dimension "d1878" = 0.5
  measures "d1876" horizontal distance of origin A0.centre
  measures "d1877" vertical distance of origin A0.centre
  measures "d1878" radius of A0
extrude "Illustrative I2C pad drill — not fabrication data" cut sketch "Sketch3 (3)" along normal blind 1.9 bodies 75 in component "Sensor / GYBMEP wired module envelope"
ref_plane "WorkPlane4" through (0, 0, 43.6) normal (0, 0, 1) x (1, 0, 0) in component "Sensor / GYBMEP wired module envelope"
sketch "Illustrative I2C plated pad sketch" plane through (0, 0, 43.6) normal (0, 0, 1) x (1, 0, 0) in component "Sensor / GYBMEP wired module envelope"
  circle A0 centre (57.2, 90.3) radius 0.85
  dimension "d1883" = 57.2
  dimension "d1884" = 90.3
  dimension "d1885" = 0.85
  measures "d1883" horizontal distance of origin A0.centre
  measures "d1884" vertical distance of origin A0.centre
  measures "d1885" radius of A0
extrude "Illustrative I2C plated pad" add sketch "Illustrative I2C plated pad sketch" along normal blind 0.08 separate body makes body 76 in component "Sensor / GYBMEP wired module envelope"
ref_plane "WorkPlane5" through (0, 0, 43.55) normal (0, 0, 1) x (1, 0, 0) in component "Sensor / GYBMEP wired module envelope"
sketch "Illustrative pad bore sketch" plane through (0, 0, 43.55) normal (0, 0, 1) x (1, 0, 0) in component "Sensor / GYBMEP wired module envelope"
  circle A0 centre (57.2, 90.3) radius 0.5
  dimension "d1890" = 57.2
  dimension "d1891" = 90.3
  dimension "d1892" = 0.5
  measures "d1890" horizontal distance of origin A0.centre
  measures "d1891" vertical distance of origin A0.centre
  measures "d1892" radius of A0
extrude "Illustrative pad bore" cut sketch "Illustrative pad bore sketch" along normal blind 0.2 bodies 76 in component "Sensor / GYBMEP wired module envelope"
ref_plane "WorkPlane6" through (0, 0, 41.9) normal (0, 0, 1) x (1, 0, 0) in component "Sensor / GYBMEP wired module envelope"
sketch "Sketch6 (2)" plane through (0, 0, 41.9) normal (0, 0, 1) x (1, 0, 0) in component "Sensor / GYBMEP wired module envelope"
  circle A0 centre (59.74, 90.3) radius 0.5
  dimension "d1897" = 59.74
  dimension "d1898" = 90.3
  dimension "d1899" = 0.5
  measures "d1897" horizontal distance of origin A0.centre
  measures "d1898" vertical distance of origin A0.centre
  measures "d1899" radius of A0
extrude "Illustrative I2C pad drill — not fabrication data (1)" cut sketch "Sketch6 (2)" along normal blind 1.9 bodies 75 in component "Sensor / GYBMEP wired module envelope"
ref_plane "WorkPlane7" through (0, 0, 43.6) normal (0, 0, 1) x (1, 0, 0) in component "Sensor / GYBMEP wired module envelope"
sketch "Illustrative I2C plated pad sketch (1)" plane through (0, 0, 43.6) normal (0, 0, 1) x (1, 0, 0) in component "Sensor / GYBMEP wired module envelope"
  circle A0 centre (59.74, 90.3) radius 0.85
  dimension "d1904" = 59.74
  dimension "d1905" = 90.3
  dimension "d1906" = 0.85
  measures "d1904" horizontal distance of origin A0.centre
  measures "d1905" vertical distance of origin A0.centre
  measures "d1906" radius of A0
extrude "Illustrative I2C plated pad (1)" add sketch "Illustrative I2C plated pad sketch (1)" along normal blind 0.08 separate body makes body 77 in component "Sensor / GYBMEP wired module envelope"
ref_plane "WorkPlane8" through (0, 0, 43.55) normal (0, 0, 1) x (1, 0, 0) in component "Sensor / GYBMEP wired module envelope"
sketch "Illustrative pad bore sketch (1)" plane through (0, 0, 43.55) normal (0, 0, 1) x (1, 0, 0) in component "Sensor / GYBMEP wired module envelope"
  circle A0 centre (59.74, 90.3) radius 0.5
  dimension "d1911" = 59.74
  dimension "d1912" = 90.3
  dimension "d1913" = 0.5
  measures "d1911" horizontal distance of origin A0.centre
  measures "d1912" vertical distance of origin A0.centre
  measures "d1913" radius of A0
extrude "Illustrative pad bore (1)" cut sketch "Illustrative pad bore sketch (1)" along normal blind 0.2 bodies 77 in component "Sensor / GYBMEP wired module envelope"
ref_plane "WorkPlane9" through (0, 0, 41.9) normal (0, 0, 1) x (1, 0, 0) in component "Sensor / GYBMEP wired module envelope"
sketch "Sketch9 (2)" plane through (0, 0, 41.9) normal (0, 0, 1) x (1, 0, 0) in component "Sensor / GYBMEP wired module envelope"
  circle A0 centre (62.28, 90.3) radius 0.5
  dimension "d1918" = 62.28
  dimension "d1919" = 90.3
  dimension "d1920" = 0.5
  measures "d1918" horizontal distance of origin A0.centre
  measures "d1919" vertical distance of origin A0.centre
  measures "d1920" radius of A0
extrude "Illustrative I2C pad drill — not fabrication data (2)" cut sketch "Sketch9 (2)" along normal blind 1.9 bodies 75 in component "Sensor / GYBMEP wired module envelope"
ref_plane "WorkPlane10" through (0, 0, 43.6) normal (0, 0, 1) x (1, 0, 0) in component "Sensor / GYBMEP wired module envelope"
sketch "Illustrative I2C plated pad sketch (2)" plane through (0, 0, 43.6) normal (0, 0, 1) x (1, 0, 0) in component "Sensor / GYBMEP wired module envelope"
  circle A0 centre (62.28, 90.3) radius 0.85
  dimension "d1925" = 62.28
  dimension "d1926" = 90.3
  dimension "d1927" = 0.85
  measures "d1925" horizontal distance of origin A0.centre
  measures "d1926" vertical distance of origin A0.centre
  measures "d1927" radius of A0
extrude "Illustrative I2C plated pad (2)" add sketch "Illustrative I2C plated pad sketch (2)" along normal blind 0.08 separate body makes body 78 in component "Sensor / GYBMEP wired module envelope"
ref_plane "WorkPlane11" through (0, 0, 43.55) normal (0, 0, 1) x (1, 0, 0) in component "Sensor / GYBMEP wired module envelope"
sketch "Illustrative pad bore sketch (2)" plane through (0, 0, 43.55) normal (0, 0, 1) x (1, 0, 0) in component "Sensor / GYBMEP wired module envelope"
  circle A0 centre (62.28, 90.3) radius 0.5
  dimension "d1932" = 62.28
  dimension "d1933" = 90.3
  dimension "d1934" = 0.5
  measures "d1932" horizontal distance of origin A0.centre
  measures "d1933" vertical distance of origin A0.centre
  measures "d1934" radius of A0
extrude "Illustrative pad bore (2)" cut sketch "Illustrative pad bore sketch (2)" along normal blind 0.2 bodies 78 in component "Sensor / GYBMEP wired module envelope"
ref_plane "WorkPlane12" through (0, 0, 41.9) normal (0, 0, 1) x (1, 0, 0) in component "Sensor / GYBMEP wired module envelope"
sketch "Sketch12" plane through (0, 0, 41.9) normal (0, 0, 1) x (1, 0, 0) in component "Sensor / GYBMEP wired module envelope"
  circle A0 centre (64.82, 90.3) radius 0.5
  dimension "d1939" = 64.82
  dimension "d1940" = 90.3
  dimension "d1941" = 0.5
  measures "d1939" horizontal distance of origin A0.centre
  measures "d1940" vertical distance of origin A0.centre
  measures "d1941" radius of A0
extrude "Illustrative I2C pad drill — not fabrication data (3)" cut sketch "Sketch12" along normal blind 1.9 bodies 75 in component "Sensor / GYBMEP wired module envelope"
ref_plane "WorkPlane13" through (0, 0, 43.6) normal (0, 0, 1) x (1, 0, 0) in component "Sensor / GYBMEP wired module envelope"
sketch "Illustrative I2C plated pad sketch (3)" plane through (0, 0, 43.6) normal (0, 0, 1) x (1, 0, 0) in component "Sensor / GYBMEP wired module envelope"
  circle A0 centre (64.82, 90.3) radius 0.85
  dimension "d1946" = 64.82
  dimension "d1947" = 90.3
  dimension "d1948" = 0.85
  measures "d1946" horizontal distance of origin A0.centre
  measures "d1947" vertical distance of origin A0.centre
  measures "d1948" radius of A0
extrude "Illustrative I2C plated pad (3)" add sketch "Illustrative I2C plated pad sketch (3)" along normal blind 0.08 separate body makes body 79 in component "Sensor / GYBMEP wired module envelope"
ref_plane "WorkPlane14" through (0, 0, 43.55) normal (0, 0, 1) x (1, 0, 0) in component "Sensor / GYBMEP wired module envelope"
sketch "Illustrative pad bore sketch (3)" plane through (0, 0, 43.55) normal (0, 0, 1) x (1, 0, 0) in component "Sensor / GYBMEP wired module envelope"
  circle A0 centre (64.82, 90.3) radius 0.5
  dimension "d1953" = 64.82
  dimension "d1954" = 90.3
  dimension "d1955" = 0.5
  measures "d1953" horizontal distance of origin A0.centre
  measures "d1954" vertical distance of origin A0.centre
  measures "d1955" radius of A0
extrude "Illustrative pad bore (3)" cut sketch "Illustrative pad bore sketch (3)" along normal blind 0.2 bodies 79 in component "Sensor / GYBMEP wired module envelope"
ref_plane "WorkPlane15" through (0, 0, 43.6) normal (0, 0, 1) x (1, 0, 0) in component "Sensor / GYBMEP wired module envelope"
sketch "Sketch15 (2)" plane through (0, 0, 43.6) normal (0, 0, 1) x (1, 0, 0) in component "Sensor / GYBMEP wired module envelope"
  line L0 (63.5, 101.5) -> (66.5, 101.5)
  line L1 (66.5, 101.5) -> (66.5, 104.5)
  line L2 (66.5, 104.5) -> (63.5, 104.5)
  line L3 (63.5, 104.5) -> (63.5, 101.5)
  dimension "d1960" = 63.5
  dimension "d1961" = 101.5
  dimension "d1962" = 3
  dimension "d1963" = 3
  constraint horizontal L0
  constraint vertical L1
  constraint horizontal L2
  constraint vertical L3
  measures "d1960" horizontal distance of origin L0.start
  measures "d1961" vertical distance of origin L0.start
  measures "d1962" horizontal distance of L0.start L0.end
  measures "d1963" vertical distance of L0.end L1.end
extrude "Humidity metal cap — placement unverified" add sketch "Sketch15 (2)" along normal blind 1.2 separate body makes body 80 in component "Sensor / GYBMEP wired module envelope"
ref_plane "WorkPlane16" through (0, 0, 43.6) normal (0, 0, 1) x (1, 0, 0) in component "Sensor / GYBMEP wired module envelope"
sketch "Regulator allocation visual sketch" plane through (0, 0, 43.6) normal (0, 0, 1) x (1, 0, 0) in component "Sensor / GYBMEP wired module envelope"
  line L0 (56.2, 94) -> (60.2, 94)
  line L1 (60.2, 94) -> (60.2, 99)
  line L2 (60.2, 99) -> (56.2, 99)
  line L3 (56.2, 99) -> (56.2, 94)
  dimension "d1968" = 56.2
  dimension "d1969" = 94
  dimension "d1970" = 4
  dimension "d1971" = 5
  constraint horizontal L0
  constraint vertical L1
  constraint horizontal L2
  constraint vertical L3
  measures "d1968" horizontal distance of origin L0.start
  measures "d1969" vertical distance of origin L0.start
  measures "d1970" horizontal distance of L0.start L0.end
  measures "d1971" vertical distance of L0.end L1.end
extrude "Regulator allocation visual" add sketch "Regulator allocation visual sketch" along normal blind 3.4 separate body makes body 81 in component "Sensor / GYBMEP wired module envelope"
ref_plane "WorkPlane17" through (0, 0, 43.6) normal (0, 0, 1) x (1, 0, 0) in component "Sensor / GYBMEP wired module envelope"
sketch "Interface IC visual sketch" plane through (0, 0, 43.6) normal (0, 0, 1) x (1, 0, 0) in component "Sensor / GYBMEP wired module envelope"
  line L0 (62, 94) -> (65, 94)
  line L1 (65, 94) -> (65, 98)
  line L2 (65, 98) -> (62, 98)
  line L3 (62, 98) -> (62, 94)
  dimension "d1976" = 62
  dimension "d1977" = 94
  dimension "d1978" = 3
  dimension "d1979" = 4
  constraint horizontal L0
  constraint vertical L1
  constraint horizontal L2
  constraint vertical L3
  measures "d1976" horizontal distance of origin L0.start
  measures "d1977" vertical distance of origin L0.start
  measures "d1978" horizontal distance of L0.start L0.end
  measures "d1979" vertical distance of L0.end L1.end
extrude "Interface IC visual" add sketch "Interface IC visual sketch" along normal blind 1.4 separate body makes body 82 in component "Sensor / GYBMEP wired module envelope"
ref_plane "WorkPlane18" through (0, 0, 43.6) normal (0, 0, 1) x (1, 0, 0) in component "Sensor / GYBMEP wired module envelope"
sketch "Passive component reference sketch" plane through (0, 0, 43.6) normal (0, 0, 1) x (1, 0, 0) in component "Sensor / GYBMEP wired module envelope"
  line L0 (58, 102.5) -> (60.5, 102.5)
  line L1 (60.5, 102.5) -> (60.5, 104)
  line L2 (60.5, 104) -> (58, 104)
  line L3 (58, 104) -> (58, 102.5)
  dimension "d1984" = 58
  dimension "d1985" = 102.5
  dimension "d1986" = 2.5
  dimension "d1987" = 1.5
  constraint horizontal L0
  constraint vertical L1
  constraint horizontal L2
  constraint vertical L3
  measures "d1984" horizontal distance of origin L0.start
  measures "d1985" vertical distance of origin L0.start
  measures "d1986" horizontal distance of L0.start L0.end
  measures "d1987" vertical distance of L0.end L1.end
extrude "Passive component reference" add sketch "Passive component reference sketch" along normal blind 0.8 separate body makes body 83 in component "Sensor / GYBMEP wired module envelope"
ref_plane "WorkPlane13" through (0, 0, 17) normal (0, 0, 1) x (1, 0, 0) in component "USB — removable panel insert and board supports"
sketch "USB flange inward corner reinforcement sketch" plane through (0, 0, 17) normal (0, 0, 1) x (1, 0, 0) in component "USB — removable panel insert and board supports"
  line L0 (69.8, 4) -> (70.7, 4)
  line L1 (70.7, 4) -> (70.7, 6.1)
  line L2 (70.7, 6.1) -> (69.8, 6.1)
  line L3 (69.8, 6.1) -> (69.8, 4)
  dimension "d2120" = 69.8
  dimension "d2121" = 4
  dimension "d2122" = 0.9
  dimension "d2123" = 2.1
  constraint horizontal L0
  constraint vertical L1
  constraint horizontal L2
  constraint vertical L3
  measures "d2120" horizontal distance of origin L0.start
  measures "d2121" vertical distance of origin L0.start
  measures "d2122" horizontal distance of L0.start L0.end
  measures "d2123" vertical distance of L0.end L1.end
extrude "USB flange inward corner reinforcement" add sketch "USB flange inward corner reinforcement sketch" along normal blind 20 bodies 37 in component "USB — removable panel insert and board supports"
ref_plane "WorkPlane14" through (0, 0, 16.9) normal (0, 0, 1) x (1, 0, 0) in component "USB — removable panel insert and board supports"
sketch "USB outside-cavity corner trim tool sketch" plane through (0, 0, 16.9) normal (0, 0, 1) x (1, 0, 0) in component "USB — removable panel insert and board supports"
  line L0 (69.7, 3.99) -> (73.2, 3.99)
  line L1 (73.2, 3.99) -> (73.2, 6)
  line L2 (73.2, 6) -> (69.7, 6)
  line L3 (69.7, 6) -> (69.7, 3.99)
  dimension "d2128" = 69.7
  dimension "d2129" = 3.99
  dimension "d2130" = 3.5
  dimension "d2131" = 2.01
  constraint horizontal L0
  constraint vertical L1
  constraint horizontal L2
  constraint vertical L3
  measures "d2128" horizontal distance of origin L0.start
  measures "d2129" vertical distance of origin L0.start
  measures "d2130" horizontal distance of L0.start L0.end
  measures "d2131" vertical distance of L0.end L1.end
extrude "USB outside-cavity corner trim tool" add sketch "USB outside-cavity corner trim tool sketch" along normal blind 20.2 separate body makes body 84 in component "USB — removable panel insert and board supports"
ref_plane "WorkPlane15" through (0, 0, 16.8) normal (0, 0, 1) x (1, 0, 0) in component "USB — removable panel insert and board supports"
sketch "Retain USB flange inside R3.50 reference sketch" plane through (0, 0, 16.8) normal (0, 0, 1) x (1, 0, 0) in component "USB — removable panel insert and board supports"
  circle A0 centre (69, 6) radius 3.5
  dimension "d2136" = 69
  dimension "d2137" = 6
  dimension "d2138" = 3.5
  measures "d2136" horizontal distance of origin A0.centre
  measures "d2137" vertical distance of origin A0.centre
  measures "d2138" radius of A0
extrude "Retain USB flange inside R3.50 reference" cut sketch "Retain USB flange inside R3.50 reference sketch" along normal blind 20.4 bodies 84 in component "USB — removable panel insert and board supports"
combine "USB flange relief follows rounded housing cavity" operation cut target body 37 tool bodies 84 in component "USB — removable panel insert and board supports"